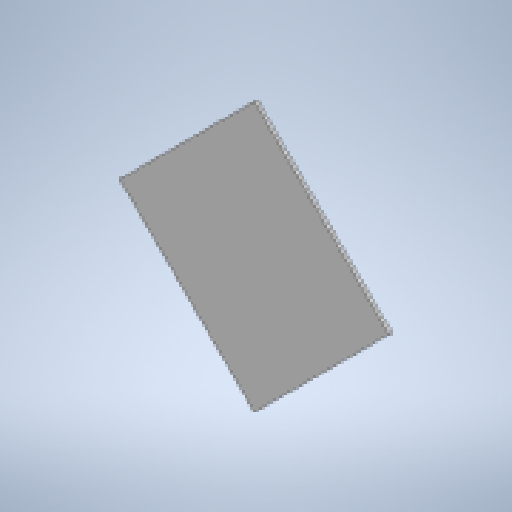
# Autodesk Inventor part: MainBase210
Saved by Autodesk Inventor 2025.1 (Build 291241000, 241)
## iProperties
Created: 2025-05-09
Part Number: MainBase210
Material: Generic
Document SubType Name: Modeling
Designer: User
Density: 1 g/cm^3
Appearance: Default
Author: User
Autodesk Inventor part; units mm, degrees
ref_plane "YZ Plane" through (0, 0, 0) normal (1, 0, 0) x (0, 1, 0)
ref_plane "XZ Plane" through (0, 0, 0) normal (0, 1, 0) x (-1, 0, 0)
ref_plane "XY Plane" through (0, 0, 0) normal (0, 0, 1) x (1, 0, 0)
sketch "Sketch1" plane through (0, 0, 0) normal (0, 0, 1) x (1, 0, 0)
  line L0 (20, 22.75) -> (-20, 22.75) projected
  line L1 (8, 74.45) -> (-8, 74.45) projected
  line L2 (0, 22.75) -> (0, 133.134)
  line L3 (28.8904, 63.2) -> (28.8904, 73.2) projected
  line L4 (28.8904, 73.2) -> (0, 102.0904)
  line L5 (28.8904, 73.2) -> (69.7476, 73.2) construction
  line L6 (0, 102.0904) -> (-36.5211, 65.5693)
  line L7 (0, 102.0904) -> (148.4924, -46.402)
  line L8 (148.4924, -46.402) -> (0, -194.8944)
  line L9 (0, -194.8944) -> (-148.4924, -46.402)
  line L10 (-148.4924, -46.402) -> (0, 102.0904)
  line L11 (0, 102.0904) -> (210, 102.0904) construction
  point P0 (0, 0)
  dimension "d0" = 135
  dimension "d1" = 90
  dimension "d2" = 210
  dimension "d3" = 45
  dimension "d4" = 210
  constraints: 18 end point, 2 equal length, 2 horizontal, 2 parallel, 1 collinear, 1 midpoint, 1 perpendicular, 1 point on line, 1 vertical
  measures "d0" angle of L5 L4
  measures "d1" angle of L6 L4
  measures "d2" distance of L4.end L7.end
  measures "d3" angle of L7 L11
  measures "d4" distance of L7.end L8.end
extrude "Extrusion1" add sketch "Sketch1" along normal blind 3.5
sketch "Sketch2" plane through (0, 0, 0) normal (0, 0, -1) x (-1, 0, 0)
  line L0 (0, 102.0904) -> (148.4924, -46.402) projected
  line L1 (-148.4924, -46.402) -> (0, 102.0904) projected
  line L2 (0, -194.8944) -> (-148.4924, -46.402) projected
  line L3 (148.4924, -46.402) -> (0, -194.8944) projected
  line L4 (-148.4924, -46.402) -> (148.4924, -46.402)
  line L5 (0, -194.8944) -> (0, 102.0904)
  circle A0 centre (0, -46.402) radius 25
  point P0 (0, 0)
  dimension "d8" = 50
  constraints: 4 end point, 1 centre point, 1 horizontal, 1 midpoint, 1 perpendicular
  measures "d8" diameter of A0
extrude "Extrusion2" cut sketch "Sketch2" against normal blind 50 contours A0 L4 L5 | L5 L4 A0 | A0 L5 L4 | L4 L5 A0
equation "\"d9\" = d8"
body "Solid1"
